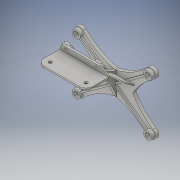
# Autodesk Inventor part: FZ6 plate bracket
Saved by Autodesk Inventor 2016 (Build 200138000, 138)
## iProperties
Created: 2016-10-14
Part Number: FZ6 plate bracket
Material: Generic
Document SubType Name: Modeling
Designer: makerspace
Density: 1 g/cm^3
Appearance: Default
Author: makerspace
Autodesk Inventor part; units mm, degrees
ref_plane "YZ Plane" through (0, 0, 0) normal (1, 0, 0) x (0, 1, 0)
ref_plane "XZ Plane" through (0, 0, 0) normal (0, 1, 0) x (-1, 0, 0)
ref_plane "XY Plane" through (0, 0, 0) normal (0, 0, 1) x (1, 0, 0)
sketch "Sketch1" plane through (0, 0, 0) normal (0, 0, 1) x (1, 0, 0)
  circle A0 centre (-69.85, 50.8) radius 9.525
  line L0 (-25.4, 19.05) -> (25.4, 19.05)
  line L1 (25.4, 19.05) -> (25.4, -19.05)
  line L2 (25.4, -19.05) -> (-25.4, -19.05)
  line L3 (-25.4, -19.05) -> (-25.4, 19.05)
  arc A1 (-62.8915, 57.3042) -> (0, 22.1446) centre (27.9812, 146.0238) ccw
  arc A2 (-34.3794, 0) -> (-73.9653, 42.2099) centre (-144.3719, -63.4873) ccw
  line L4 (0, 71.4969) -> (0, -47.1844) construction
  circle A3 centre (69.85, 50.8) radius 9.525
  arc A4 (0, 22.1446) -> (62.8915, 57.3042) centre (-27.9812, 146.0238) ccw
  arc A5 (73.9653, 42.2099) -> (34.3794, 0) centre (144.3719, -63.4873) ccw
  line L5 (-104.8988, 0) -> (91.0292, 0) construction
  circle A6 centre (-69.85, -50.8) radius 9.525
  arc A7 (0, -22.1446) -> (-62.8915, -57.3042) centre (27.9812, -146.0238) ccw
  arc A8 (-73.9653, -42.2099) -> (-34.3794, 0) centre (-144.3719, 63.4873) ccw
  circle A9 centre (69.85, -50.8) radius 9.525
  arc A10 (62.8915, -57.3042) -> (0, -22.1446) centre (-27.9812, -146.0238) ccw
  arc A11 (34.3794, 0) -> (73.9653, -42.2099) centre (144.3719, 63.4873) ccw
  point P0 (0, 0)
  point P1 (0, 19.05)
  point P2 (-25.4, 0)
  dimension "d0" = 19.05
  dimension "d1" = 69.85
  dimension "d2" = 50.8
  dimension "d3" = 50.8
  dimension "d4" = 38.1
  dimension "d5" = 127
  dimension "d6" = 127
  constraints: 24 point on circle, 16 symmetric about line, 12 centre point, 12 end point, 3 point on line, 2 horizontal, 2 midpoint, 2 parallel, 1 horizontal alignment, 1 perpendicular, 1 vertical, 1 vertical alignment, 9 other
  measures "d0" diameter of A0
  measures "d1" horizontal distance of point (0, 0) A0.centre
  measures "d2" vertical distance of point (0, 0) A0.centre
  measures "d3" distance of L0.start L0.end
  measures "d4" distance of L2.end L0.start
  measures "d5" radius of A1
  measures "d6" radius of A2
extrude "Extrusion1" add sketch "Sketch1" along normal blind 6.35 contours A0 | A0 A1 A4 A3 A5 A11 A9 A10 A7 A6 A8 A2 | A3 | A6 | A9 | L0 L1 L2 L3
sketch "Sketch2" plane through (0, 0, 6.35) normal (0, 0, 1) x (1, 0, 0)
  arc A0 (-73.9653, -42.2099) -> (-62.8915, -57.3042) centre (-69.85, -50.8) ccw projected
  arc A1 (0, -22.1446) -> (-62.8915, -57.3042) centre (27.9812, -146.0238) ccw projected
  arc A2 (62.8915, -57.3042) -> (0, -22.1446) centre (-27.9812, -146.0238) ccw projected
  arc A3 (62.8915, -57.3042) -> (73.9653, -42.2099) centre (69.85, -50.8) ccw projected
  arc A4 (34.3794, 0) -> (73.9653, -42.2099) centre (144.3719, 63.4873) ccw projected
  arc A5 (73.9653, 42.2099) -> (34.3794, 0) centre (144.3719, -63.4873) ccw projected
  arc A6 (73.9653, 42.2099) -> (62.8915, 57.3042) centre (69.85, 50.8) ccw projected
  arc A7 (0, 22.1446) -> (62.8915, 57.3042) centre (-27.9812, 146.0238) ccw projected
  arc A8 (-62.8915, 57.3042) -> (0, 22.1446) centre (27.9812, 146.0238) ccw projected
  arc A9 (-62.8915, 57.3042) -> (-73.9653, 42.2099) centre (-69.85, 50.8) ccw projected
  arc A10 (-34.3794, 0) -> (-73.9653, 42.2099) centre (-144.3719, -63.4873) ccw projected
  arc A11 (-73.9653, -42.2099) -> (-34.3794, 0) centre (-144.3719, 63.4873) ccw projected
  circle A12 centre (-69.85, 50.8) radius 7.9375
  circle A13 centre (69.85, 50.8) radius 7.9375
  circle A14 centre (-69.85, -50.8) radius 7.9375
  circle A15 centre (69.85, -50.8) radius 7.9375
  point P0 (0, 0)
  dimension "d9" = 15.875
  dimension "d10" = 15.875
  dimension "d11" = 15.875
  dimension "d12" = 15.875
  constraints: 4 centre point, 4 coincident
  measures "d9" diameter of A12
  measures "d10" diameter of A13
  measures "d11" diameter of A14
  measures "d12" diameter of A15
extrude "Extrusion2" add sketch "Sketch2" along normal blind 6.35 contours A12 | A13 | A14 | A15
sketch "Sketch3" plane through (-69.85, 50.8, 12.7) normal (0, 0, 1) x (1, 0, 0)
  circle A0 centre (0, 0) radius 7.9375 projected
  circle A1 centre (139.7, 0) radius 7.9375 projected
  circle A2 centre (139.7, -101.6) radius 7.9375 projected
  circle A3 centre (0, -101.6) radius 7.9375 projected
  circle A4 centre (0, 0) radius 4.7625 construction
  line L0 (2.7496, 4.7625) -> (5.4993, 0)
  line L1 (5.4993, 0) -> (2.7496, -4.7625)
  line L2 (2.7496, -4.7625) -> (-2.7496, -4.7625)
  line L3 (-2.7496, -4.7625) -> (-5.4993, 0)
  line L4 (-5.4993, 0) -> (-2.7496, 4.7625)
  line L5 (-2.7496, 4.7625) -> (2.7496, 4.7625)
  line L6 (0, 0) -> (139.7, 0) construction
  line L7 (0, 0) -> (0, -101.6) construction
  line L8 (134.2007, 0) -> (136.9504, 4.7625)
  line L9 (136.9504, 4.7625) -> (142.4496, 4.7625)
  line L10 (142.4496, 4.7625) -> (145.1993, 0)
  line L11 (145.1993, 0) -> (142.4496, -4.7625)
  line L12 (142.4496, -4.7625) -> (136.9504, -4.7625)
  line L13 (136.9504, -4.7625) -> (134.2007, 0)
  line L14 (-5.4993, -101.6) -> (-2.7496, -96.8375)
  line L15 (-2.7496, -96.8375) -> (2.7496, -96.8375)
  line L16 (2.7496, -96.8375) -> (5.4993, -101.6)
  line L17 (5.4993, -101.6) -> (2.7496, -106.3625)
  line L18 (2.7496, -106.3625) -> (-2.7496, -106.3625)
  line L19 (-2.7496, -106.3625) -> (-5.4993, -101.6)
  line L20 (134.2007, -101.6) -> (136.9504, -96.8375)
  line L21 (136.9504, -96.8375) -> (142.4496, -96.8375)
  line L22 (142.4496, -96.8375) -> (145.1993, -101.6)
  line L23 (145.1993, -101.6) -> (142.4496, -106.3625)
  line L24 (142.4496, -106.3625) -> (136.9504, -106.3625)
  line L25 (136.9504, -106.3625) -> (134.2007, -101.6)
  point P0 (69.85, -50.8)
  point P1 (0, 4.7625)
  point P2 (139.7, 4.7625)
  point P3 (0, -96.8375)
  point P4 (139.7, -96.8375)
  dimension "d15" = 9.525
  dimension "d20" = 139.7
  dimension "d23" = 101.6
  constraints: 52 end point, 2 coincident, 2 horizontal, 2 vertical, 1 midpoint, 1 vertical alignment, 54 other
  measures "d20" distance of L3.end L8.start
  measures "d23" distance of L3.end L14.start
extrude "Extrusion3" cut sketch "Sketch3" against normal blind 6.35 contours L0 L1 L2 L3 L4 L5 | L8 L9 L10 L11 L12 L13 | L14 L15 L16 L17 L18 L19 | L20 L21 L22 L23 L24 L25
sketch "Sketch4" plane through (-69.85, 50.8, 6.35) normal (0, 0, 1) x (1, 0, 0)
  line L0 (-2.7496, 4.7625) -> (2.7496, 4.7625) projected
  line L1 (2.7496, 4.7625) -> (5.4993, 0) projected
  line L2 (5.4993, 0) -> (2.7496, -4.7625) projected
  line L3 (2.7496, -4.7625) -> (-2.7496, -4.7625) projected
  line L4 (-2.7496, -4.7625) -> (-5.4993, 0) projected
  line L5 (-5.4993, 0) -> (-2.7496, 4.7625) projected
  circle A0 centre (0, 0) radius 7.9375 projected
  circle A1 centre (139.7, 0) radius 7.9375 projected
  line L6 (2.7496, -106.3625) -> (-2.7496, -106.3625) projected
  line L7 (-2.7496, -106.3625) -> (-5.4993, -101.6) projected
  line L8 (-5.4993, -101.6) -> (-2.7496, -96.8375) projected
  line L9 (-2.7496, -96.8375) -> (2.7496, -96.8375) projected
  line L10 (2.7496, -96.8375) -> (5.4993, -101.6) projected
  line L11 (5.4993, -101.6) -> (2.7496, -106.3625) projected
  circle A2 centre (0, -101.6) radius 7.9375 projected
  circle A3 centre (139.7, -101.6) radius 7.9375 projected
  circle A4 centre (0, 0) radius 2.3813
  circle A5 centre (139.7, 0) radius 2.3813
  circle A6 centre (0, -101.6) radius 2.3813
  circle A7 centre (139.7, -101.6) radius 2.3813
  point P0 (69.85, -50.8)
  dimension "d26" = 4.7625
  dimension "d27" = 4.7625
  dimension "d28" = 4.7625
  dimension "d29" = 4.7625
  constraints: 4 centre point, 4 coincident
  measures "d26" diameter of A4
  measures "d27" diameter of A5
  measures "d28" diameter of A6
  measures "d29" diameter of A7
extrude "Extrusion4" cut sketch "Sketch4" against normal through all contours A4 | A5 | A6 | A7
sketch "Sketch5" plane through (0, 0, 6.35) normal (0, 0, 1) x (1, 0, 0)
  circle A0 centre (-69.85, -50.8) radius 7.9375 projected
  circle A1 centre (-69.85, 50.8) radius 7.9375 projected
  circle A2 centre (69.85, 50.8) radius 7.9375 projected
  circle A3 centre (69.85, -50.8) radius 7.9375 projected
  arc A4 (-73.9653, -42.2099) -> (-62.8915, -57.3042) centre (-69.85, -50.8) ccw projected
  arc A5 (0, -22.1446) -> (-62.8915, -57.3042) centre (27.9812, -146.0238) ccw projected
  arc A6 (62.8915, -57.3042) -> (0, -22.1446) centre (-27.9812, -146.0238) ccw projected
  arc A7 (62.8915, -57.3042) -> (73.9653, -42.2099) centre (69.85, -50.8) ccw projected
  arc A8 (34.3794, 0) -> (73.9653, -42.2099) centre (144.3719, 63.4873) ccw projected
  arc A9 (73.9653, 42.2099) -> (34.3794, 0) centre (144.3719, -63.4873) ccw projected
  arc A10 (73.9653, 42.2099) -> (62.8915, 57.3042) centre (69.85, 50.8) ccw projected
  arc A11 (0, 22.1446) -> (62.8915, 57.3042) centre (-27.9812, 146.0238) ccw projected
  arc A12 (-62.8915, 57.3042) -> (0, 22.1446) centre (27.9812, 146.0238) ccw projected
  arc A13 (-62.8915, 57.3042) -> (-73.9653, 42.2099) centre (-69.85, 50.8) ccw projected
  arc A14 (-34.3794, 0) -> (-73.9653, 42.2099) centre (-144.3719, -63.4873) ccw projected
  arc A15 (-73.9653, -42.2099) -> (-34.3794, 0) centre (-144.3719, 63.4873) ccw projected
  line L0 (-69.85, 50.8) -> (69.85, -50.8) construction
  line L1 (69.85, 50.8) -> (-69.85, -50.8) construction
  line L2 (-64.4941, 44.9418) -> (-2.699, 0)
  line L3 (0, -1.9629) -> (62.6266, -47.5096)
  line L4 (62.6266, 47.5096) -> (0, 1.9629)
  line L5 (-2.699, 0) -> (-64.4941, -44.9418)
  line L6 (64.4941, -44.9418) -> (2.699, 0)
  line L7 (0, 1.9629) -> (-62.6266, 47.5096)
  line L8 (-62.6266, -47.5096) -> (0, -1.9629)
  line L9 (2.699, 0) -> (64.4941, 44.9418)
  point P0 (0, 0)
  point P1 (0, 0)
  point P2 (0, 0)
  constraints: 24 end point, 8 parallel, 8 point on circle, 2 midpoint
extrude "Extrusion5" add sketch "Sketch5" along normal blind 3.175 contours A0 L5 L2 A1 L7 L4 A2 L9 L6 A3 L3 L8
sketch "Sketch6" plane through (0, 0, 0) normal (1, 0, 0) x (0, 1, 0)
  line L0 (0, 0) -> (63.5, 0)
  line L1 (63.5, 101.6) -> (0, 101.6)
  line L2 (22.1446, 6.35) -> (-22.1446, 6.35)
  line L3 (63.5, 66.675) -> (73.7666, 70.9276)
  arc A0 (73.7666, 70.9276) -> (22.1446, 6.35) centre (141.754, -36.3418) ccw
  arc A1 (-22.1446, 6.35) -> (63.5, 101.6) centre (-60.8722, 127.3011) ccw
  line L4 (0, 101.6) -> (0, 15.84)
  line L5 (0, 6.35) -> (0, 0)
  line L6 (63.5, 0) -> (63.5, 63.6848)
  line L7 (63.5, 66.675) -> (63.5, 101.6)
  dimension "d37" = 63.5
  dimension "d38" = 101.6
  dimension "d39" = 11.1125
  dimension "d41" = 34.925
  dimension "d44" = 127
  dimension "d45" = 127
  constraints: 16 end point, 6 point on circle, 5 parallel, 2 centre point, 2 horizontal, 2 perpendicular, 1 midpoint
  measures "d37" distance of L1.end L1.start
  measures "d38" distance of L1.start L0.end
  measures "d39" distance of L3.start L3.end
  measures "d41" distance of L1.start L3.start
  measures "d44" radius of A0
  measures "d45" radius of A1
extrude "Extrusion6" add sketch "Sketch6" along normal mid plane 6.35 contours L2 A1 L7 L3 A0
sketch "Sketch9" plane through (-3.175, 63.5, 101.6) normal (0, 1, 0) x (1, 0, 0)
  line L0 (25.4, 3.6382) -> (38.1, 3.6382) construction
  line L1 (-31.75, -9.0618) -> (38.1, -9.0618)
  arc A0 (-44.45, 3.6382) -> (-31.75, -9.0618) centre (-31.75, 3.6382) ccw
  arc A1 (38.1, -9.0618) -> (50.8, 3.6382) centre (38.1, 3.6382) ccw
  line L2 (25.4, 3.6382) -> (50.8, 3.6382) construction
  line L3 (50.8, 3.6382) -> (50.8, 34.925)
  line L4 (50.8, 34.925) -> (-44.45, 34.925)
  line L5 (-44.45, 34.925) -> (-44.45, 3.6382)
  point P0 (3.175, 101.6)
  point P1 (3.175, 3.6382)
  point P2 (6.35, 34.925)
  dimension "d52" = 34.925
  dimension "d53" = 25.4
  dimension "d54" = 34.925
  constraints: 13 end point, 5 point on circle, 2 centre point, 2 horizontal, 2 parallel, 2 point on line, 2 tangent, 1 perpendicular
  measures "d52" distance of point (3.175, 3.638) L0.end
  measures "d53" diameter of A1
  measures "d54" distance of point (3.175, 3.638) A0.centre
extrude "Extrusion7" add sketch "Sketch9" against normal blind 3.175
sketch "Sketch10" plane through (-3.175, 73.7666, 70.9276) normal (0, -0.3826834, 0.9238795) x (1, 0, 0)
  line L0 (-26.9875, 0.2753) -> (33.3375, 0.2753) construction
  arc A0 (-33.4141, 7.3056) -> (-35.2609, 4.9951) centre (-26.9875, 0.2753) ccw
  arc A1 (41.6109, 4.9951) -> (39.7641, 7.3056) centre (33.3375, 0.2753) ccw
  line L1 (50.8, -11.1125) -> (-44.45, -11.1125)
  line L2 (-44.45, -11.1125) -> (-35.2609, 4.9951)
  line L3 (50.8, -11.1125) -> (41.6109, 4.9951)
  line L4 (39.7641, 7.3056) -> (-33.4141, 7.3056)
  point P0 (3.175, -95.2943)
  point P1 (3.175, 0.2753)
  dimension "d57" = 30.1625
  dimension "d58" = 19.05
  constraints: 12 end point, 4 point on circle, 3 horizontal, 2 centre point, 2 tangent, 1 midpoint
  measures "d57" distance of point (3.175, 0.275) L0.end
  measures "d58" diameter of A1
extrude "Extrusion8" add sketch "Sketch10" against normal blind 3.175
sketch "Sketch11" plane through (0, 0, 0) normal (1, 0, 0) x (0, 1, 0)
  line L0 (63.5, 66.675) -> (60.325, 66.675) projected
  line L1 (63.5, 66.675) -> (64.715, 63.7417) projected
  line L2 (60.325, 66.675) -> (64.715, 63.7417)
  line L3 (63.5, 66.675) -> (60.325, 66.675)
  point P0 (0, 0)
  constraints: 4 end point, 1 horizontal
extrude "Extrusion9" add sketch "Sketch11" along normal mid plane 95.25
sketch "Sketch12" plane through (-3.175, 74.9816, 67.9943) normal (0, 0.3826834, -0.9238795) x (-1, 0, 0)
  arc A0 (-39.7641, 7.3056) -> (-41.6109, 4.9951) centre (-33.3375, 0.2753) ccw projected
  arc A1 (35.2609, 4.9951) -> (33.4141, 7.3056) centre (26.9875, 0.2753) ccw projected
  circle A2 centre (-33.3375, 0.2753) radius 9.525
  circle A3 centre (26.9875, 0.2753) radius 9.525
  line L0 (33.4141, 7.3056) -> (-39.7641, 7.3056) projected
  line L1 (-39.7641, 7.3056) -> (-26.9109, 7.3056)
  point P0 (-3.175, -95.2943)
  dimension "d83" = 19.05
  dimension "d64" = 19.05
  constraints: 2 coincident, 2 end point, 1 centre point, 1 point on line, 3 other
  measures "d64" diameter of A3
extrude "Extrusion10" add sketch "Sketch12" along normal blind 3.175
sketch "Sketch13" plane through (30.1625, 76.451, 65.1663) normal (0, 0.3826834, -0.9238795) x (-1, 0, 0)
  circle A0 centre (0, 0) radius 9.525 projected
  circle A1 centre (60.325, 0) radius 9.525 projected
  circle A2 centre (0, 0) radius 3.175
  circle A3 centre (60.325, 0) radius 3.175
  point P0 (30.1625, -95.5696)
  dimension "d67" = 6.35
  dimension "d68" = 6.35
  constraints: 2 centre point, 2 coincident
  measures "d67" diameter of A2
  measures "d68" diameter of A3
extrude "Extrusion11" cut sketch "Sketch13" against normal up to next contours A2 | A3
sketch "Sketch14" plane through (-3.175, 60.325, 101.6) normal (0, -1, 0) x (1, 0, 0)
  arc A0 (50.8, -3.6382) -> (38.1, 9.0618) centre (38.1, -3.6382) ccw projected
  arc A1 (-31.75, 9.0618) -> (-44.45, -3.6382) centre (-31.75, -3.6382) ccw projected
  circle A2 centre (38.1, -3.6382) radius 9.525
  circle A3 centre (-31.75, -3.6382) radius 9.525
  point P0 (3.175, -101.6)
  dimension "d71" = 19.05
  dimension "d72" = 19.05
  constraints: 2 centre point, 2 coincident
  measures "d71" diameter of A2
  measures "d72" diameter of A3
extrude "Extrusion12" add sketch "Sketch14" along normal blind 3.175
sketch "Sketch15" plane through (34.925, 57.15, 97.9618) normal (0, -1, 0) x (1, 0, 0)
  circle A0 centre (0, 0) radius 9.525 projected
  circle A1 centre (-69.85, 0) radius 9.525 projected
  circle A2 centre (0, 0) radius 6.35
  circle A3 centre (-69.85, 0) radius 6.35
  point P0 (-34.925, -97.9618)
  dimension "d75" = 12.7
  dimension "d76" = 12.7
  constraints: 2 centre point, 2 coincident
  measures "d75" diameter of A2
  measures "d76" diameter of A3
extrude "Extrusion13" cut sketch "Sketch15" against normal blind 3.175 contours A2 | A3
sketch "Sketch16" plane through (34.925, 60.325, 97.9618) normal (0, -1, 0) x (1, 0, 0)
  circle A0 centre (0, 0) radius 6.35 projected
  circle A1 centre (-69.85, 0) radius 6.35 projected
  circle A2 centre (0, 0) radius 3.175
  circle A3 centre (-69.85, 0) radius 3.175
  point P0 (-34.925, -97.9618)
  dimension "d79" = 6.35
  dimension "d80" = 6.35
  constraints: 2 centre point, 2 coincident
  measures "d79" diameter of A2
  measures "d80" diameter of A3
extrude "Extrusion14" cut sketch "Sketch16" against normal through all contours A2 | A3
sketch "Sketch17" plane through (30.1625, 76.451, 65.1663) normal (0, 0.3826834, -0.9238795) x (-1, 0, 0)
  circle A0 centre (0, 0) radius 3.175 projected
  circle A1 centre (0, 0) radius 9.525 projected
  circle A2 centre (60.325, 0) radius 3.175 projected
  circle A3 centre (60.325, 0) radius 9.525 projected
  circle A4 centre (0, 0) radius 6.35
  circle A5 centre (60.325, 0) radius 6.35
  point P0 (30.1625, -95.5696)
  dimension "d84" = 12.7
  dimension "d85" = 12.7
  constraints: 2 centre point, 2 coincident
  measures "d84" diameter of A4
  measures "d85" diameter of A5
extrude "Extrusion15" cut sketch "Sketch17" against normal blind 3.175 contours A4 | A5
ref_plane "Work Plane2" through (3.175, 38.9756, 38.2612) normal (0, 0.8092783, -0.5874255) x (-1, 0, 0)
sketch "Sketch18" plane through (3.175, 38.9756, 38.2612) normal (0, 0.8092783, -0.5874255) x (-1, 0, 0)
  line L0 (0, 35.5358) -> (-44.45, 35.5358) projected
  line L1 (6.35, 35.7121) -> (0, 35.7121) projected
  line L2 (0, -35.7121) -> (0, 35.7121) projected
  line L3 (3.175, -35.7121) -> (0, -35.7121) projected
  line L4 (6.35, -35.7121) -> (3.175, -35.7121) projected
  line L5 (6.35, 35.7121) -> (6.35, -35.7121) projected
  line L6 (50.8, 35.5358) -> (6.35, 35.5358) projected
  ellipse E0 centre (31.1562, 37.0577) end of major axis (-95.8438, 37.0577) minor radius 74.603 (-59.7165, -15.0584) -> (3.175, -35.7121) ccw projected
  ellipse E1 centre (-24.8062, 37.0577) end of major axis (-151.8062, 37.0577) minor radius 74.603 (3.175, -35.7121) -> (66.0665, -15.0584) ccw projected
  arc A0 (22.225, 3.2239) -> (41.275, -17.3979) centre (124.4658, 78.5619) ccw
  arc A1 (50.8, 35.5358) -> (22.225, 3.2239) centre (130.2658, -63.5308) ccw
  arc A2 (6.4547, -35.2499) -> (6.35, -35.7121) centre (130.2658, -63.5308) ccw
  line L7 (3.175, -40.851) -> (3.175, -35.7121) projected
  line L8 (6.35, -43.6414) -> (65.8016, -18.2426) projected
  line L9 (-59.4516, -18.2426) -> (0, -43.6414) projected
  line L10 (41.275, -41.785) -> (41.275, -17.3979)
  arc A3 (-34.925, -17.3979) -> (-15.875, 3.2239) centre (-118.1158, 78.5619) ccw
  arc A4 (-15.875, 3.2239) -> (-44.45, 35.5358) centre (-123.9158, -63.5308) ccw
  line L11 (-34.925, -41.785) -> (-34.925, -17.3979)
  line L12 (0, -35.7121) -> (0, 35.7121) projected
  line L13 (-34.925, -41.785) -> (41.275, -41.785)
  line L14 (-44.45, 35.5358) -> (50.8, 35.5358)
  point P0 (3.175, -53.8593)
  point P1 (49.0598, -23.6288)
  dimension "d88" = 127
  dimension "d90" = 38.1
  dimension "d91" = 19.05
  constraints: 10 point on circle, 8 end point, 5 centre point, 5 symmetric about line, 2 horizontal, 1 vertical, 6 other
  measures "d88" radius of A0
  measures "d90" distance between parallel lines of L7 L10
  measures "d91" distance from line of L7 A0.start
extrude "Extrusion16" add sketch "Sketch18" against normal blind 1.5875 contours L2 E0 L11 A3 A4 L0 | L2 L3 L4 A2 E1 L10 L8 L13 L9 L11 E0 | L6 A1 A0 L10 E1 L5 | E1 A2 L5 | L9 L13 L11 | L8 L10 L13
sketch "Sketch20" plane through (0, 0, 0) normal (1, 0, 0) x (0, 1, 0)
  line L0 (59.8503, 67.0196) -> (58.5655, 67.9521) projected
  arc A0 (64.1009, 64.152) -> (38.9756, 38.2612) centre (141.754, -36.3418) ccw projected
  line L1 (60.325, 66.675) -> (60.325, 97.9618) projected
  line L2 (58.5655, 67.9521) -> (60.325, 70.3761)
  line L3 (60.325, 70.3761) -> (60.325, 66.675)
  line L4 (60.325, 66.675) -> (64.1009, 64.152)
  line L5 (59.8503, 67.0196) -> (56.1201, 61.8807)
  line L6 (56.1201, 61.8807) -> (64.1009, 64.152)
  line L7 (58.5655, 67.9521) -> (59.8503, 67.0196)
  line L8 (60.325, 70.3761) -> (60.325, 66.675)
  point P0 (0, 0)
  dimension "d96" = 6.35
  constraints: 14 end point, 2 vertical, 1 collinear, 1 perpendicular, 1 point on line
  measures "d96" distance of L0.start L5.end
extrude "Extrusion17" add sketch "Sketch20" along normal mid plane 76.2
chamfer "Chamfer1" distance 1.5875 distance2 3.175 1 edges at (-30.1625, 84.0359, 71.7447) measured on face at (-30.1625, 82.4994, 71.1082)
chamfer "Chamfer2" distance 1.5875 distance2 3.175 1 edges at (30.1625, 84.0359, 71.7447)
equation "\"d54\" = d52"
equation "\"d64\" = d63"
equation "\"d63\" = 19.05"
body "Solid1"
